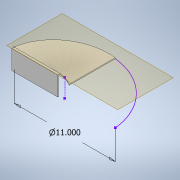
# Autodesk Inventor part: ramp
Saved by Autodesk Inventor 2020 (Build 240168000, 168)
## iProperties
Created: 2021-03-23
Part Number: ramp
Material: Generic
Document SubType Name: Modeling
Designer: tdmp4
Density: 1 g/cm^3
Appearance: Default
Author: tdmp4
Autodesk Inventor part; units mm, degrees
ref_plane "YZ Plane" through (0, 0, 0) normal (1, 0, 0) x (0, 1, 0)
ref_plane "XZ Plane" through (0, 0, 0) normal (0, 1, 0) x (-1, 0, 0)
ref_plane "XY Plane" through (0, 0, 0) normal (0, 0, 1) x (1, 0, 0)
sketch "Sketch6" plane through (0, 0, 0) normal (0, 0, 1) x (1, 0, 0)
  line L0 (139.7, -0.0309) -> (12.7, -0.0309)
  line L1 (12.7, -0.0309) -> (12.7, 2.5091)
  line L2 (12.7, 2.5091) -> (139.7, 2.5091)
  line L3 (139.7, 2.5091) -> (139.7, -0.0309)
  point P0 (0, 0)
  dimension "d11" = 127
  dimension "d12" = 2.54
  constraints: 8 end point, 2 parallel, 1 horizontal, 1 perpendicular
  measures "d11" distance of L1.end L2.end
  measures "d12" distance of L0.end L1.end
sketch3d "3D Sketch2"
  helix H0 starts at (139.7, 0, 0) axis through (0, 0, 0) along (0, 1, 0) pitch 101.6 turns 0.5 hand right
sweep "Sweep1" add profiles "Sketch6" path "3D Sketch2"
ref_plane "Work Plane1" through (-139.7, 53.3091, 0) normal (0, 1, 0) x (-1, 0, 0)
sketch "Sketch13" plane through (-139.7, 53.3091, 0) normal (0, 1, 0) x (-1, 0, 0)
  line L0 (-139.7, 0) -> (-304.3793, 0)
  line L1 (-304.3793, 0) -> (-304.3793, -146.5732)
  line L2 (-304.3793, -146.5732) -> (-139.7, -146.5732)
  line L3 (-139.7, -146.5732) -> (-139.7, 0)
  constraints: 8 end point, 2 parallel, 1 horizontal, 1 perpendicular
extrude "Extrusion6" cut sketch "Sketch13" against normal blind 138.1125
sketch "Sketch14" plane through (-139.7, 53.3091, 0) normal (0, 0, 1) x (1, 0, 0)
  line L0 (0, -2.54) -> (127, -2.54) projected
  line L1 (127, -2.54) -> (0, -2.54)
  line L2 (0, -2.54) -> (0, 0)
  line L3 (0, 0) -> (127, 0)
  line L4 (127, 0) -> (127, -2.54)
  point P0 (139.7, -53.3091)
  constraints: 8 end point, 2 parallel, 1 horizontal, 1 perpendicular
extrude "Extrusion7" add sketch "Sketch14" along normal blind 6.35
sketch "Sketch15" plane through (-139.7, 50.7691, 0) normal (0, -1, 0) x (1, 0, 0)
  line L0 (0, 0) -> (0, 6.35) projected
  line L1 (127, 0) -> (127, 6.35) projected
  line L2 (0, 6.35) -> (127, 6.35)
  line L3 (127, 6.35) -> (127, 3.81)
  line L4 (127, 3.81) -> (0, 3.81)
  line L5 (0, 3.81) -> (0, 6.35)
  point P0 (139.7, 0)
  point P1 (0, 3.81)
  dimension "d38" = 2.54
  constraints: 8 end point, 2 parallel, 1 horizontal, 1 perpendicular, 1 point on line
  measures "d38" distance of L2.end L3.end
extrude "Extrusion8" add sketch "Sketch15" along normal blind 50.8
body "Solid1"
